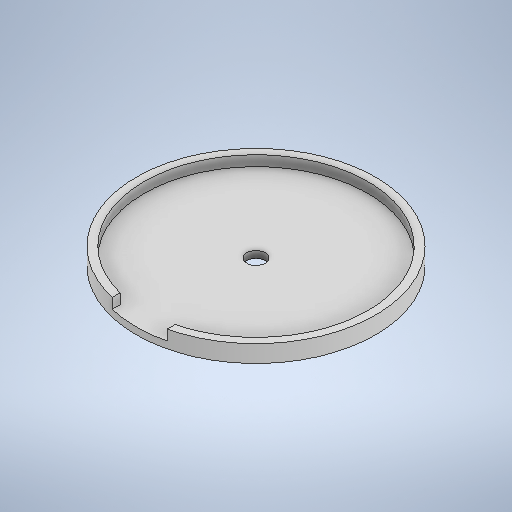
# Autodesk Inventor part: 2024_08_28_Holder_disk_NMR
Saved by Autodesk Inventor 2025.1 (Build 291241000, 241)
## iProperties
Created: 2024-08-28
Part Number: 2024_08_28_Holder_disk_NMR
Material: Generisch
Document SubType Name: Modeling
Designer: to86hug
Density: 1 g/cm^3
Appearance: Vorgabe
Author: to86hug
Autodesk Inventor part; units mm, degrees
ref_plane "YZ Plane" through (0, 0, 0) normal (1, 0, 0) x (0, 1, 0)
ref_plane "XZ Plane" through (0, 0, 0) normal (0, 1, 0) x (-1, 0, 0)
ref_plane "XY Plane" through (0, 0, 0) normal (0, 0, 1) x (1, 0, 0)
sketch "Skizze1" plane through (0, 0, 0) normal (0, 0, 1) x (1, 0, 0)
  circle A0 centre (0, 0) radius 34.775
  dimension "d0" = 69.55
  constraints: 1 centre point, 1 coincident
  measures "d0" diameter of A0
extrude "Extrusion1" add sketch "Skizze1" along normal blind 5
sketch "Skizze2" plane through (0, 0, 5) normal (0, 0, 1) x (1, 0, 0)
  circle A0 centre (0, 0) radius 32.54
  dimension "d3" = 65.08
  constraints: 1 centre point, 1 coincident
  measures "d3" diameter of A0
extrude "Extrusion2" cut sketch "Skizze2" against normal blind 3
sketch "Skizze3" plane through (0, 0, 0) normal (0, 0, -1) x (-1, 0, 0)
  circle A0 centre (0, 0) radius 2.69
  dimension "d6" = 5.38
  constraints: 1 centre point, 1 coincident
  measures "d6" diameter of A0
extrude "Extrusion3" cut sketch "Skizze3" against normal through all
sketch "Skizze4" plane through (0, 0, 5) normal (0, 0, 1) x (1, 0, 0)
  line L0 (-8, -42.775) -> (8, -42.775)
  line L1 (8, -42.775) -> (8, -26.775)
  line L2 (8, -26.775) -> (-8, -26.775)
  line L3 (-8, -26.775) -> (-8, -42.775)
  circle A0 centre (0, 0) radius 34.775 projected
  line L4 (-8, -42.775) -> (8, -26.775) construction
  line L5 (8, -42.775) -> (-8, -26.775) construction
  point P0 (0, -34.775)
  dimension "d9" = 16
  dimension "d10" = 16
  constraints: 12 end point, 2 midpoint, 2 parallel, 1 horizontal, 1 perpendicular, 1 vertical alignment, 1 other
  measures "d9" distance of L2.end L1.end
  measures "d10" distance of L1.end L0.end
extrude "Extrusion4" cut sketch "Skizze4" against normal up to surface (3 mm away) contours L3 A0 L1 L0 | L3 L2 L1 A0 picked at (0.896, -29.407)
